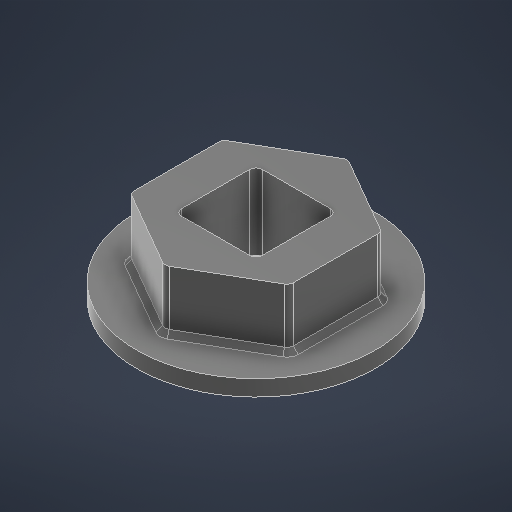
# Autodesk Inventor part: insert
Saved by Autodesk Inventor 2025.2 (Build 292293000, 293)
## iProperties
Created: 2026-01-16
Part Number: insert
Material: Acetal Resin, Black
Document SubType Name: Modeling
Designer: cloudy
Density: 1.425 g/cm^3
Appearance: Smooth - Black
Author: cloudy
Autodesk Inventor part; units mm, degrees
ref_plane "YZ Plane" through (0, 0, 0) normal (1, 0, 0) x (0, 1, 0)
ref_plane "XZ Plane" through (0, 0, 0) normal (0, 1, 0) x (-1, 0, 0)
ref_plane "XY Plane" through (0, 0, 0) normal (0, 0, 1) x (1, 0, 0)
sketch "Sketch1" plane through (0, 0, 0) normal (0, 1, 0) x (-1, 0, 0)
  circle A0 centre (0, 0) radius 9.525
  dimension "d0" = 19.05
  constraints: 1 centre point, 1 coincident
  measures "d0" diameter of A0
extrude "Extrusion1" add sketch "Sketch1" along normal blind 1.27
sketch "Sketch2" plane through (0, 1.27, 0) normal (0, 1, 0) x (1, 0, 0)
  line L0 (6.35, -3.6662) -> (0, -7.3323)
  line L1 (0, -7.3323) -> (-6.35, -3.6662)
  line L2 (-6.35, -3.6662) -> (-6.35, 3.6662)
  line L3 (-6.35, 3.6662) -> (0, 7.3323)
  line L4 (0, 7.3323) -> (6.35, 3.6662)
  line L5 (6.35, 3.6662) -> (6.35, -3.6662)
  point P0 (0, 0)
  point P1 (0, 0)
  dimension "d4" = 12.7
  constraints: 12 end point, 1 coincident, 1 vertical, 13 other
  measures "d4" distance between parallel lines of L5 L2
extrude "Extrusion2" add sketch "Sketch2" along normal blind 4.7625
fillet "Fillet1" radius 0.508 6 edges at (6.35, 3.6513, 3.6662) (6.35, 3.6513, -3.6662) (0, 3.6513, -7.3323) (0, 3.6513, 7.3323) (-6.35, 3.6513, 3.6662) (-6.35, 3.6513, -3.6662)
sketch "Sketch3" plane through (0, 6.0325, 0) normal (0, 1, 0) x (1, 0, 0)
  line L0 (-2.7178, -3.2258) -> (2.7178, -3.2258)
  line L1 (3.2258, -2.7178) -> (3.2258, 2.7178)
  line L2 (2.7178, 3.2258) -> (-2.7178, 3.2258)
  line L3 (-3.2258, 2.7178) -> (-3.2258, -2.7178)
  line L4 (-3.2258, -3.2258) -> (3.2258, 3.2258) construction
  line L5 (3.2258, -3.2258) -> (-3.2258, 3.2258) construction
  arc A0 (-3.2258, -2.7178) -> (-2.7178, -3.2258) centre (-2.7178, -2.7178) ccw
  arc A1 (2.7178, -3.2258) -> (3.2258, -2.7178) centre (2.7178, -2.7178) ccw
  arc A2 (3.2258, 2.7178) -> (2.7178, 3.2258) centre (2.7178, 2.7178) ccw
  arc A3 (-2.7178, 3.2258) -> (-3.2258, 2.7178) centre (-2.7178, 2.7178) ccw
  point P0 (0, 0)
  dimension "d8" = 6.4516
  dimension "d9" = 0.508
  constraints: 12 end point, 8 point on circle, 8 point on line, 8 tangent, 4 centre point, 3 equal radius, 2 midpoint, 2 parallel, 2 perpendicular, 1 horizontal
  measures "d8" distance of L4.end L5.end
  measures "d9" radius of A0
extrude "Extrusion3" cut sketch "Sketch3" against normal through all
chamfer "Chamfer1" distance 0.3969 angle 45 12 edges at (3.175, 1.27, -5.4993) (6.2819, 1.27, -3.6269) (6.35, 1.27, 0) (6.2819, 1.27, 3.6269) (3.175, 1.27, 5.4993) (0, 1.27, 7.2538) (-3.175, 1.27, 5.4993) (-6.2819, 1.27, 3.6269) (-6.35, 1.27, 0) (-6.2819, 1.27, -3.6269) (-3.175, 1.27, -5.4993) (0, 1.27, -7.2538)
body "Solid1"
